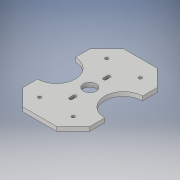
# Autodesk Inventor part: motor mount plate
Saved by Autodesk Inventor 2019 (Build 230136000, 136)
## iProperties
Created: 2023-11-01
Part Number: motor mount plate
Material: Generic
Document SubType Name: Modeling
Designer: ony
Density: 1 g/cm^3
Appearance: Default
Author: ony
Autodesk Inventor part; units mm, degrees
ref_plane "YZ Plane" through (0, 0, 0) normal (1, 0, 0) x (0, 1, 0)
ref_plane "XZ Plane" through (0, 0, 0) normal (0, 1, 0) x (-1, 0, 0)
ref_plane "XY Plane" through (0, 0, 0) normal (0, 0, 1) x (1, 0, 0)
sketch "Sketch1" plane through (0, 0, 0) normal (0, 1, 0) x (-1, 0, 0)
  line L0 (-0.2028, 19.4) -> (-0.2028, 32.1) construction
  line L1 (-2.584, 19.4) -> (-2.584, 32.1)
  line L2 (2.1785, 32.1) -> (2.1785, 19.4)
  arc A0 (-2.584, 19.4) -> (2.1785, 19.4) centre (-0.2028, 19.4) ccw
  arc A1 (2.1785, 32.1) -> (-2.584, 32.1) centre (-0.2028, 32.1) ccw
  line L3 (-0.2028, -19.4) -> (-0.2028, -32.1) construction
  line L4 (-2.584, -19.4) -> (-2.584, -32.1)
  line L5 (2.1785, -32.1) -> (2.1785, -19.4)
  arc A2 (2.1785, -19.4) -> (-2.584, -19.4) centre (-0.2028, -19.4) ccw
  arc A3 (-2.584, -32.1) -> (2.1785, -32.1) centre (-0.2028, -32.1) ccw
  line L6 (-51.0028, -76.2) -> (50.5972, -76.2)
  line L7 (50.5972, -76.2) -> (50.5972, 76.2)
  line L8 (50.5972, 76.2) -> (-51.0028, 76.2)
  line L9 (-51.0028, 76.2) -> (-51.0028, -76.2)
  line L10 (-51.0028, -76.2) -> (50.5972, 76.2) construction
  line L11 (50.5972, -76.2) -> (-51.0028, 76.2) construction
  line L12 (50.5972, 76.2) -> (50.5972, 50.8)
  line L13 (50.5972, 50.8) -> (25.1972, 50.8)
  line L14 (-51.0028, 76.2) -> (-51.0028, 50.8)
  line L15 (-51.0028, 50.8) -> (-25.6028, 50.8)
  line L16 (50.5972, -76.2) -> (50.5972, -50.8)
  line L17 (50.5972, -50.8) -> (25.1972, -50.8)
  line L18 (-51.0028, -76.2) -> (-51.0028, -50.8)
  line L19 (-51.0028, -50.8) -> (-25.6028, -50.8)
  circle A4 centre (25.1972, 50.8) radius 2.3813
  circle A5 centre (25.1972, -50.8) radius 2.3812
  circle A6 centre (-25.6028, 50.8) radius 2.3812
  circle A7 centre (-25.6028, -50.8) radius 2.3812
  arc A8 (-2.584, 31.6606) -> (-2.584, -31.6606) centre (-0.2028, 0) ccw
  arc A9 (2.1785, -31.6606) -> (2.1785, 31.6606) centre (-0.2028, 0) ccw
  point P0 (0, 0)
  dimension "d7" = 101.6
  dimension "d8" = 152.4
  dimension "d9" = 25.4
  dimension "d10" = 25.4
  dimension "d11" = 25.4
  dimension "d12" = 25.4
  dimension "d13" = 25.4
  dimension "d14" = 25.4
  dimension "d15" = 25.4
  dimension "d16" = 25.4
  dimension "d17" = 4.7625
  dimension "d18" = 4.7625
  dimension "d19" = 4.7625
  dimension "d20" = 4.7625
  constraints: 44 end point, 12 point on circle, 10 centre point, 8 point on line, 8 tangent, 5 perpendicular, 4 coincident, 4 parallel, 2 midpoint, 1 horizontal
  measures "d7" distance of L8.end L7.end
  measures "d8" distance of L7.end L6.end
  measures "d9" distance of L7.end L12.end
  measures "d10" distance of L12.end L13.end
  measures "d11" distance of L8.end L14.end
  measures "d12" distance of L14.end L15.end
  measures "d13" distance of L6.end L16.end
  measures "d14" distance of L16.end L17.end
  measures "d15" distance of L6.start L18.end
  measures "d16" distance of L18.end L19.end
  measures "d17" diameter of A4
  measures "d18" diameter of A5
  measures "d19" diameter of A6
  measures "d20" diameter of A7
extrude "Extrusion1" add sketch "Sketch1" along normal blind 6.35 contours A0 L2 A9 L5 A2 L4 A8 L1 | L9 L8 L7 L6
sketch "Sketch2" plane through (0, 6.35, 0) normal (0, 1, 0) x (1, 0, 0)
  circle A0 centre (0, 0) radius 9.75
  dimension "d23" = 19.5
  constraints: 1 centre point, 1 coincident
  measures "d23" diameter of A0
extrude "Extrusion2" cut sketch "Sketch2" against normal blind 6.35
sketch "Sketch3" plane through (0, 6.35, 0) normal (0, 1, 0) x (1, 0, 0)
  line L0 (-6.6401, -37.7246) -> (10.2278, -37.7246)
  line L1 (10.2278, -37.7246) -> (10.2278, -15.7747)
  line L2 (10.2278, -15.7747) -> (-6.6401, -15.7747)
  line L3 (-6.6401, -15.7747) -> (-6.6401, -37.7246)
  line L4 (-9.2351, 15.4742) -> (5.254, 15.4742)
  line L5 (5.254, 15.4742) -> (5.254, 41.8573)
  line L6 (5.254, 41.8573) -> (-9.2351, 41.8573)
  line L7 (-9.2351, 41.8573) -> (-9.2351, 15.4742)
  point P0 (0, 0)
  constraints: 16 end point, 4 parallel, 2 horizontal, 2 perpendicular
extrude "Extrusion3" add sketch "Sketch3" against normal blind 6.35
sketch "Sketch4" plane through (0, 6.35, 0) normal (0, 1, 0) x (1, 0, 0)
  circle A0 centre (0, 0) radius 31.75
  line L0 (0, -31.75) -> (0, -25.75)
  line L1 (0, 31.75) -> (0, 25.75)
  circle A1 centre (0, -25.75) radius 2.3812
  circle A2 centre (0, 25.75) radius 2.3813
  line L2 (0, -22.75) -> (0, -28.75) construction
  line L3 (2.3812, -22.75) -> (2.3812, -28.75)
  line L4 (-2.3812, -28.75) -> (-2.3812, -22.75)
  arc A3 (2.3812, -22.75) -> (-2.3812, -22.75) centre (0, -22.75) ccw
  arc A4 (-2.3812, -28.75) -> (2.3812, -28.75) centre (0, -28.75) ccw
  line L5 (0, 22.75) -> (0, 28.75) construction
  line L6 (2.3813, 22.75) -> (2.3813, 28.75)
  line L7 (-2.3813, 28.75) -> (-2.3813, 22.75)
  arc A5 (-2.3813, 22.75) -> (2.3813, 22.75) centre (0, 22.75) ccw
  arc A6 (2.3813, 28.75) -> (-2.3813, 28.75) centre (0, 28.75) ccw
  dimension "d28" = 63.5
  dimension "d29" = 6
  dimension "d30" = 6
  dimension "d31" = 4.7625
  dimension "d32" = 4.7625
  constraints: 20 end point, 10 point on circle, 8 tangent, 7 centre point, 4 midpoint, 3 coincident, 2 parallel, 2 vertical
  measures "d28" diameter of A0
  measures "d29" distance of L0.start L0.end
  measures "d30" distance of L1.start L1.end
  measures "d31" diameter of A1
  measures "d32" diameter of A2
extrude "Extrusion4" cut sketch "Sketch4" against normal blind 6.35 contours A6 L6 A2 L1 | L1 A2 L7 A6 | A4 L4 A1 L0 | L0 A1 L3 A4 | A2 | A1 | L6 A5 L7 A2 | L4 A3 L3 A1
chamfer "Chamfer1" distance 25.4 angle 45 4 edges at (-50.5972, 3.175, 76.2) (51.0028, 3.175, 76.2) (-50.5972, 3.175, -76.2) (51.0028, 3.175, -76.2)
sketch "Sketch5" plane through (0, 6.35, 0) normal (0, 1, 0) x (1, 0, 0)
  line L0 (-50.5972, 50.8) -> (-50.5972, -50.8) projected
  circle A0 centre (-50.5972, 0) radius 28.575
  line L1 (51.0028, -50.8) -> (51.0028, 50.8) projected
  circle A1 centre (51.0028, 0) radius 28.575
  point P0 (0, 0)
  dimension "d38" = 57.15
  dimension "d39" = 57.15
  constraints: 2 centre point, 2 midpoint
  measures "d38" diameter of A0
  measures "d39" diameter of A1
extrude "Extrusion5" cut sketch "Sketch5" against normal blind 6.35
body "Solid1"
